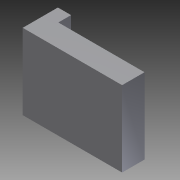
# Autodesk Inventor part: lid_f
Saved by Autodesk Inventor 2011 (Build 150239000, 239)
## iProperties
Created: 2011-05-24
Part Number: lid_f
Document SubType Name: Modeling
Designer: labuser
Density: 1 g/cm^3
Author: labuser
Autodesk Inventor part; units mm, degrees
ref_plane "YZ Plane" through (0, 0, 0) normal (1, 0, 0) x (0, 1, 0)
ref_plane "XZ Plane" through (0, 0, 0) normal (0, 1, 0) x (-1, 0, 0)
ref_plane "XY Plane" through (0, 0, 0) normal (0, 0, 1) x (1, 0, 0)
sketch "Sketch1" plane through (0, 0, 0) normal (0, 0, 1) x (1, 0, 0)
  line L0 (0, 0) -> (5.8, 0) construction
  line L1 (5.8, 0) -> (5.8, 4.3) construction
  line L2 (5.8, 4.3) -> (0, 4.3) construction
  line L3 (0, 4.3) -> (0, 0) construction
  line L4 (5.8, 4.3) -> (-5.5, 4.3)
  line L5 (-5.5, 4.3) -> (-5.5, -4.3)
  line L6 (-5.5, -4.3) -> (5.8, -4.3)
  line L7 (5.8, -4.3) -> (5.8, 4.3)
  dimension "d0" = 5.8
  dimension "d1" = 4.3
  dimension "d2" = 11.3
  dimension "d3" = 8.6
  constraints: 16 end point, 4 parallel, 2 horizontal, 2 perpendicular
  measures "d0" distance of L2.end L1.end
  measures "d1" distance of L1.end L0.end
  measures "d2" distance of L6.end L5.end
  measures "d3" distance of L5.end L4.end
extrude "Extrusion1" add sketch "Sketch1" along normal blind 4
sketch "Sketch2" plane through (0, 0, 0) normal (0, 0, -1) x (-1, 0, 0)
  line L0 (-5.8, 4.3) -> (5.5, 4.3) projected
  line L1 (5.5, -4.3) -> (4, -4.3) construction
  line L2 (4, -4.3) -> (4, 4.3) construction
  line L3 (4, 4.3) -> (5.5, 4.3) construction
  line L4 (5.5, 4.3) -> (5.5, -4.3) construction
  line L5 (4, -4.3) -> (-5.8, -4.3)
  line L6 (-5.8, -4.3) -> (-5.8, 4.3)
  line L7 (-5.8, 4.3) -> (4, 4.3)
  line L8 (4, 4.3) -> (4, -4.3)
  point P0 (0, 0)
  dimension "d6" = 1.5
  constraints: 16 end point, 4 parallel, 2 horizontal, 2 perpendicular, 1 point on line
  measures "d6" distance of L2.end L3.end
extrude "Extrusion2" cut sketch "Sketch2" against normal blind 1.45
sketch "Sketch3" plane through (0, 0, 1.45) normal (0, 0, -1) x (-1, 0, 0)
  line L0 (4, -4.3) -> (4, 4.3) projected
  line L1 (-5.8, -4.3) -> (-5.4, -4.3) construction
  line L2 (-5.4, -4.3) -> (-5.4, -3.9) construction
  line L3 (-5.4, -3.9) -> (-5.8, -3.9) construction
  line L4 (-5.8, -3.9) -> (-5.8, -4.3) construction
  line L5 (-5.8, 4.3) -> (-5.4, 4.3) construction
  line L6 (-5.4, 4.3) -> (-5.4, 3.9) construction
  line L7 (-5.4, 3.9) -> (-5.8, 3.9) construction
  line L8 (-5.8, 3.9) -> (-5.8, 4.3) construction
  line L9 (-5.4, -3.9) -> (4, -3.9)
  line L10 (4, -3.9) -> (4, 3.9)
  line L11 (4, 3.9) -> (-5.4, 3.9)
  line L12 (-5.4, 3.9) -> (-5.4, -3.9)
  point P0 (0, 0)
  dimension "d9" = 0.4
  dimension "d10" = 0.4
  dimension "d11" = 0.4
  dimension "d12" = 0.4
  constraints: 24 end point, 6 parallel, 3 horizontal, 3 perpendicular, 1 point on line
  measures "d9" distance of L3.end L2.end
  measures "d10" distance of L2.end L1.end
  measures "d11" distance of L6.end L7.end
  measures "d12" distance of L5.end L6.end
extrude "Extrusion3" cut sketch "Sketch3" against normal blind 0.8
body "Solid1"
